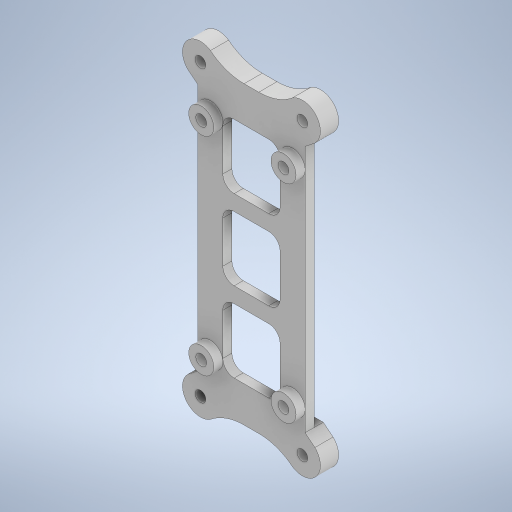
# Autodesk Inventor part: Flight Controller Mount
Saved by Autodesk Inventor 2023 (Build 270158000, 158)
## iProperties
Created: 2022-11-05
Part Number: Flight Controller Mount
Material: Generic
Document SubType Name: Modeling
Designer: mjlangfo
Density: 1 g/cm^3
Appearance: Default
Author: mjlangfo
Autodesk Inventor part; units mm, degrees
ref_plane "YZ Plane" through (0, 0, 0) normal (1, 0, 0) x (0, 1, 0)
ref_plane "XZ Plane" through (0, 0, 0) normal (0, 1, 0) x (-1, 0, 0)
ref_plane "XY Plane" through (0, 0, 0) normal (0, 0, 1) x (1, 0, 0)
sketch "Sketch1" plane through (0, 0, 0) normal (0, 0, 1) x (1, 0, 0)
  line L0 (28.2876, 87.8245) -> (13.6204, 76.0012) projected
  arc A0 (28.2876, 87.8245) -> (28.7404, 92.0429) centre (26.4048, 90.1602) ccw construction
  line L1 (26.2301, 95.1571) -> (28.7404, 92.0429) construction
  arc A1 (26.2301, 95.1571) -> (22.0117, 95.61) centre (23.8944, 93.2744) ccw construction
  line L2 (11.4653, 87.1085) -> (22.0117, 95.61) construction
  arc A2 (2.0515, 83.7867) -> (11.4653, 87.1085) centre (2.0515, 98.7867) ccw projected
  line L3 (-2.0515, 83.7867) -> (2.0515, 83.7867) projected
  arc A3 (-11.4653, 87.1085) -> (-2.0515, 83.7867) centre (-2.0515, 98.7867) ccw projected
  line L4 (-22.0117, 95.61) -> (-11.4653, 87.1085) construction
  arc A4 (-22.0117, 95.61) -> (-26.2301, 95.1571) centre (-23.8944, 93.2744) ccw construction
  line L5 (-28.7404, 92.0429) -> (-26.2301, 95.1571) construction
  arc A5 (-28.7404, 92.0429) -> (-28.2876, 87.8245) centre (-26.4048, 90.1602) ccw construction
  line L6 (-13.6204, 76.0012) -> (-28.2876, 87.8245) projected
  arc A6 (-13.6204, 76.0012) -> (-7.3445, 73.7867) centre (-7.3445, 83.7867) ccw construction
  line L7 (7.3445, 73.7867) -> (-7.3445, 73.7867) projected
  arc A7 (7.3445, 73.7867) -> (13.6204, 76.0012) centre (7.3445, 83.7867) ccw construction
  circle A8 centre (-23.5925, 90.4621) radius 1.475 construction
  circle A9 centre (23.5925, 90.4621) radius 1.475 construction
  circle A10 centre (-14.25, 82.931) radius 1.475 projected
  circle A11 centre (14.25, 82.931) radius 1.475 projected
  line L8 (28.2876, -2.9109) -> (13.6204, 8.9124) projected
  arc A12 (13.6204, 8.9124) -> (7.3445, 11.127) centre (7.3445, 1.127) ccw construction
  line L9 (7.3445, 11.127) -> (-7.3445, 11.127) projected
  arc A13 (-7.3445, 11.127) -> (-13.6204, 8.9124) centre (-7.3445, 1.127) ccw construction
  line L10 (-13.6204, 8.9124) -> (-28.2876, -2.9109) projected
  arc A14 (-28.2876, -2.9109) -> (-28.7404, -7.1293) centre (-26.4048, -5.2465) ccw construction
  line L11 (-28.7404, -7.1293) -> (-26.2301, -10.2435) construction
  arc A15 (-26.2301, -10.2435) -> (-22.0117, -10.6963) centre (-23.8944, -8.3607) ccw construction
  line L12 (-22.0117, -10.6963) -> (-11.4653, -2.1949) construction
  arc A16 (-2.0515, 1.127) -> (-11.4653, -2.1949) centre (-2.0515, -13.873) ccw projected
  line L13 (-2.0515, 1.127) -> (2.0515, 1.127) projected
  arc A17 (11.4653, -2.1949) -> (2.0515, 1.127) centre (2.0515, -13.873) ccw projected
  line L14 (11.4653, -2.1949) -> (22.0117, -10.6963) construction
  arc A18 (22.0117, -10.6963) -> (26.2301, -10.2435) centre (23.8944, -8.3607) ccw construction
  line L15 (26.2301, -10.2435) -> (28.7404, -7.1293) construction
  arc A19 (28.7404, -7.1293) -> (28.2876, -2.9109) centre (26.4048, -5.2465) ccw construction
  circle A20 centre (-23.5925, -5.5484) radius 1.475 construction
  circle A21 centre (23.5925, -5.5484) radius 1.475 construction
  circle A22 centre (-14.25, 1.9826) radius 1.475 projected
  circle A23 centre (14.25, 1.9826) radius 1.475 projected
  arc A24 (10.926, -1.78) -> (17.0347, 6.1601) centre (14.25, 1.9826) ccw
  line L16 (-8, 79.2868) -> (-15, 79.2868) construction
  line L17 (-15, 79.2868) -> (-15, 77.1134)
  line L18 (-15, 5.6268) -> (-8, 5.6268) construction
  line L19 (-8, 14.302) -> (-8, 25.952)
  line L20 (15, 79.2868) -> (8, 79.2868) construction
  line L21 (8, 70.6117) -> (8, 58.9617)
  line L22 (8, 5.6268) -> (15, 5.6268) construction
  line L23 (15, 5.6268) -> (15, 7.8003)
  arc A25 (17.0347, 6.1601) -> (10.926, -1.78) centre (14.25, 1.9826) ccw construction
  arc A26 (17.0347, 78.7535) -> (10.926, 86.6936) centre (14.25, 82.931) ccw
  arc A27 (-10.926, 86.6936) -> (-17.0347, 78.7535) centre (-14.25, 82.931) ccw
  arc A28 (-11.4653, -2.1949) -> (-17.7412, 5.5906) centre (-14.25, 1.9826) ccw construction
  arc A29 (10.926, 86.6936) -> (17.0347, 78.7535) centre (14.25, 82.931) ccw construction
  arc A30 (-17.0347, 78.7535) -> (-10.926, 86.6936) centre (-14.25, 82.931) ccw construction
  arc A31 (-17.7412, 5.5906) -> (-11.4653, -2.1949) centre (-14.25, 1.9826) ccw
  line L24 (0, 73.7867) -> (4.825, 73.7867)
  line L25 (0, 73.7867) -> (-4.825, 73.7867)
  line L26 (0, 11.127) -> (4.825, 11.127)
  line L27 (0, 11.127) -> (-4.825, 11.127)
  arc A32 (8, 70.6117) -> (4.825, 73.7867) centre (4.825, 70.6117) ccw
  arc A33 (-4.825, 73.7867) -> (-8, 70.6117) centre (-4.825, 70.6117) ccw
  arc A34 (4.825, 11.127) -> (8, 14.302) centre (4.825, 14.302) ccw
  arc A35 (-8, 14.302) -> (-4.825, 11.127) centre (-4.825, 14.302) ccw
  line L28 (-15, 77.1134) -> (-15, 7.8003)
  line L29 (-15, 7.8003) -> (-15, 5.6268)
  line L30 (15, 7.8003) -> (15, 77.1134)
  line L31 (15, 77.1134) -> (15, 79.2868)
  line L32 (4.825, 55.7867) -> (-4.825, 55.7867)
  line L33 (-8, 55.7867) -> (-8, 51.4568) construction
  line L34 (-4.825, 51.4568) -> (4.825, 51.4568)
  line L35 (8, 51.4568) -> (8, 55.7867)
  line L36 (4.825, 33.4568) -> (-4.825, 33.4568)
  line L37 (-8, 33.4568) -> (-8, 29.127) construction
  line L38 (-4.825, 29.127) -> (4.825, 29.127)
  line L39 (8, 29.127) -> (8, 33.4568) construction
  line L40 (8, 55.7867) -> (8, 51.4568) construction
  line L41 (8, 48.2818) -> (8, 36.6318)
  line L42 (-8, 58.9617) -> (-8, 70.6117)
  line L43 (-8, 51.4568) -> (-8, 55.7867)
  line L44 (-8, 36.6318) -> (-8, 48.2818)
  line L45 (-8, 29.127) -> (-8, 33.4568)
  line L46 (8, 33.4568) -> (8, 29.127)
  line L47 (8, 25.952) -> (8, 14.302)
  arc A36 (4.825, 55.7867) -> (8, 58.9617) centre (4.825, 58.9617) ccw
  arc A37 (-8, 58.9617) -> (-4.825, 55.7867) centre (-4.825, 58.9617) ccw
  arc A38 (8, 48.2818) -> (4.825, 51.4568) centre (4.825, 48.2818) ccw
  arc A39 (-4.825, 51.4568) -> (-8, 48.2818) centre (-4.825, 48.2818) ccw
  arc A40 (-8, 36.6318) -> (-4.825, 33.4568) centre (-4.825, 36.6318) ccw
  arc A41 (4.825, 33.4568) -> (8, 36.6318) centre (4.825, 36.6318) ccw
  arc A42 (8, 25.952) -> (4.825, 29.127) centre (4.825, 25.952) ccw
  arc A43 (-4.825, 29.127) -> (-8, 25.952) centre (-4.825, 25.952) ccw
  point P0 (0, 0)
  point P1 (0, 1.127)
  point P2 (0, 83.7867)
  point P3 (8, 73.8082)
  point P4 (15, 73.7867)
  point P5 (-15, 73.7867)
  point P6 (15, 11.127)
  point P7 (-15, 11.127)
  point P8 (-17.7412, 79.3231)
  point P9 (17.7412, 5.5906)
  point P10 (17.7412, 79.3231)
  point P11 (-4.825, 73.7867)
  point P12 (4.825, 73.7867)
  point P13 (4.825, 11.127)
  point P14 (-4.825, 11.127)
  point P15 (0, 33.4568)
  dimension "d0" = 7
  dimension "d1" = 7
  dimension "d2" = 73.66
  dimension "d5" = 4.4999
  dimension "d6" = 4.4999
  dimension "d9" = 3.175
  dimension "d10" = 3.175
  dimension "d16" = 30
  dimension "d17" = 15
  dimension "d32" = 18
  dimension "d33" = 18
  dimension "d34" = 18
  dimension "d35" = 4.3299
  dimension "d36" = 4.3299
  dimension "d37" = 3.175
  constraints: 64 end point, 49 point on line, 48 point on circle, 40 tangent, 36 parallel, 20 centre point, 10 perpendicular, 9 equal radius, 5 midpoint, 4 coincident, 3 horizontal
  measures "d0" distance of L20.start L20.end
  measures "d1" distance of L16.start L16.end
  measures "d2" distance of L18.end L16.start
  measures "d5" distance between parallel lines of L3 L20
  measures "d6" distance between parallel lines of L13 L22
  measures "d9" radius of A32
  measures "d10" radius of A34
  measures "d16" distance between parallel lines of L28 L30
  measures "d17" distance from line of point (0, 83.787) L28
  measures "d32" distance between parallel lines of L32 L24
  measures "d33" distance from line of point (0, 33.457) L34
  measures "d34" distance between parallel lines of L26 L38
  measures "d35" distance between parallel lines of L34 L32
  measures "d36" distance between parallel lines of L38 L36
  measures "d37" radius of A36
extrude "Extrusion1" add sketch "Sketch1" along normal blind 2.54 contours L0 L30 L8 A24 A17 L13 A16 A31 L10 L28 L6 A27 A3 L3 A2 A26
sketch "Sketch2" plane through (0, 0, 2.54) normal (0, 0, 1) x (1, 0, 0)
  line L0 (2.0515, 83.7867) -> (-2.0515, 83.7867) projected
  line L1 (-2.0515, 1.127) -> (2.0515, 1.127) projected
  line L2 (15, 7.8003) -> (15, 77.1134) projected
  line L3 (-15, 77.1134) -> (-15, 7.8003) projected
  circle A0 centre (11.5, 71.4568) radius 3.5
  circle A1 centre (11.5, 13.4568) radius 3.5
  circle A2 centre (-11.5, 13.4568) radius 3.5
  circle A3 centre (-11.5, 71.4568) radius 3.5
  point P0 (0, 0)
  point P1 (0, 83.7867)
  point P2 (0, 83.7867)
  point P3 (0, 83.7867)
  point P4 (0, 1.127)
  dimension "d13" = 7
  dimension "d14" = 58
  dimension "d15" = 23
  dimension "d18" = 7
  dimension "d19" = 7
  dimension "d20" = 7
  dimension "d22" = 23
  dimension "d23" = 58
  dimension "d24" = 11.5
  dimension "d27" = 12.3299
  dimension "d29" = 12.3299
  constraints: 4 centre point, 4 midpoint, 1 horizontal alignment, 1 vertical alignment
  measures "d13" diameter of A0
  measures "d14" distance of A1.centre A0.centre
  measures "d15" distance of A2.centre A1.centre
  measures "d18" diameter of A1
  measures "d19" diameter of A2
  measures "d20" diameter of A3
  measures "d22" distance of A3.centre A0.centre
  measures "d23" distance of A2.centre A3.centre
  measures "d24" horizontal distance of point (0, 83.787) A0.centre
  measures "d27" distance from line of L0 A0.centre
  measures "d29" distance from line of L1 A1.centre
extrude "Extrusion2" add sketch "Sketch2" along normal blind 2.54
sketch "Sketch3" plane through (-11.5, 71.4568, 5.08) normal (0, 0, 1) x (1, 0, 0)
  circle A0 centre (23, 0) radius 3.5 projected
  circle A1 centre (0, 0) radius 3.5 projected
  circle A2 centre (0, -58) radius 3.5 projected
  circle A3 centre (23, -58) radius 3.5 projected
  circle A4 centre (23, 0) radius 1.5
  circle A5 centre (0, 0) radius 1.5
  circle A6 centre (0, -58) radius 1.5
  circle A7 centre (23, -58) radius 1.5
  point P0 (11.5, -71.4568)
  dimension "d38" = 3
  dimension "d39" = 3
  dimension "d40" = 3
  dimension "d41" = 3
  constraints: 4 centre point, 4 coincident
  measures "d38" diameter of A4
  measures "d39" diameter of A5
  measures "d40" diameter of A6
  measures "d41" diameter of A7
extrude "Extrusion3" cut sketch "Sketch3" against normal up to next contours A4 | A5 | A6 | A7
sketch "Sketch4" plane through (0, 0, 0) normal (0, 0, -1) x (-1, 0, 0)
  line L0 (-15, 71.4568) -> (-15, 77.1134) projected
  line L1 (15, 77.1134) -> (-15, 77.1134)
  line L2 (15, 77.1134) -> (15, 7.8003) projected
  line L3 (-17.7412, 5.5906) -> (-15, 7.8003) projected
  line L4 (15, 7.8003) -> (-15, 7.8003)
  circle A0 centre (11.5, 13.4568) radius 1.5 projected
  circle A1 centre (-11.5, 13.4568) radius 1.5 projected
  circle A2 centre (11.5, 71.4568) radius 1.5 projected
  circle A3 centre (-11.5, 71.4568) radius 1.5 projected
  arc A4 (2.0515, 83.7867) -> (11.4653, 87.1085) centre (2.0515, 98.7867) ccw projected
  line L5 (-2.0515, 83.7867) -> (2.0515, 83.7867) projected
  arc A5 (-11.4653, 87.1085) -> (-2.0515, 83.7867) centre (-2.0515, 98.7867) ccw projected
  arc A6 (-11.4653, 87.1085) -> (-17.7412, 79.3231) centre (-14.25, 82.931) ccw projected
  line L6 (-15, 77.1134) -> (-17.7412, 79.3231) projected
  line L7 (-15, 7.8003) -> (-15, 77.1134) projected
  line L8 (-17.7412, 5.5906) -> (-15, 7.8003) projected
  arc A7 (-17.7412, 5.5906) -> (-11.4653, -2.1949) centre (-14.25, 1.9826) ccw projected
  arc A8 (-2.0515, 1.127) -> (-11.4653, -2.1949) centre (-2.0515, -13.873) ccw projected
  line L9 (2.0515, 1.127) -> (-2.0515, 1.127) projected
  arc A9 (11.4653, -2.1949) -> (2.0515, 1.127) centre (2.0515, -13.873) ccw projected
  arc A10 (11.4653, -2.1949) -> (17.7412, 5.5906) centre (14.25, 1.9826) ccw projected
  line L10 (15, 7.8003) -> (17.7412, 5.5906) projected
  line L11 (15, 77.1134) -> (15, 7.8003) projected
  line L12 (17.7412, 79.3231) -> (15, 77.1134) projected
  arc A11 (17.7412, 79.3231) -> (11.4653, 87.1085) centre (14.25, 82.931) ccw projected
  line L13 (8, 14.302) -> (8, 25.952) projected
  arc A12 (4.825, 11.127) -> (8, 14.302) centre (4.825, 14.302) ccw projected
  line L14 (-4.825, 11.127) -> (4.825, 11.127) projected
  arc A13 (-8, 14.302) -> (-4.825, 11.127) centre (-4.825, 14.302) ccw projected
  line L15 (-8, 25.952) -> (-8, 14.302) projected
  arc A14 (-4.825, 29.127) -> (-8, 25.952) centre (-4.825, 25.952) ccw projected
  line L16 (4.825, 29.127) -> (-4.825, 29.127) projected
  arc A15 (8, 25.952) -> (4.825, 29.127) centre (4.825, 25.952) ccw projected
  line L17 (-8, 70.6117) -> (-8, 58.9617) projected
  arc A16 (-4.825, 73.7867) -> (-8, 70.6117) centre (-4.825, 70.6117) ccw projected
  line L18 (4.825, 73.7867) -> (-4.825, 73.7867) projected
  arc A17 (8, 70.6117) -> (4.825, 73.7867) centre (4.825, 70.6117) ccw projected
  line L19 (8, 58.9617) -> (8, 70.6117) projected
  arc A18 (4.825, 55.7867) -> (8, 58.9617) centre (4.825, 58.9617) ccw projected
  line L20 (-4.825, 55.7867) -> (4.825, 55.7867) projected
  arc A19 (-8, 58.9617) -> (-4.825, 55.7867) centre (-4.825, 58.9617) ccw projected
  line L21 (8, 36.6318) -> (8, 48.2818) projected
  arc A20 (4.825, 33.4568) -> (8, 36.6318) centre (4.825, 36.6318) ccw projected
  line L22 (-4.825, 33.4568) -> (4.825, 33.4568) projected
  arc A21 (-8, 36.6318) -> (-4.825, 33.4568) centre (-4.825, 36.6318) ccw projected
  line L23 (-8, 48.2818) -> (-8, 36.6318) projected
  arc A22 (-4.825, 51.4568) -> (-8, 48.2818) centre (-4.825, 48.2818) ccw projected
  line L24 (4.825, 51.4568) -> (-4.825, 51.4568) projected
  arc A23 (8, 48.2818) -> (4.825, 51.4568) centre (4.825, 48.2818) ccw projected
  circle A24 centre (-14.25, 1.9826) radius 1.475 projected
  circle A25 centre (14.25, 1.9826) radius 1.475 projected
  circle A26 centre (-14.25, 82.931) radius 1.475 projected
  circle A27 centre (14.25, 82.931) radius 1.475 projected
  point P0 (0, 0)
  point P1 (-17.7412, 5.5906)
  constraints: 4 end point, 2 horizontal
extrude "Extrusion4" add sketch "Sketch4" along normal blind 2.54 contours L6 A6 A5 L5 A4 A11 L12 L1 | L4 L10 A10 A9 L9 A8 A7 L3
equation "\"d1\" = d0"
equation "\"d5\" = d6"
equation "\"d17\" = 0.5 * d16"
equation "\"d32\" = d33"
equation "\"d34\" = d33"
equation "\"d35\" = d36"
equation "\"d18\" = d13"
equation "\"d19\" = d13"
equation "\"d20\" = d13"
equation "\"d22\" = d15"
equation "\"d23\" = d14"
equation "\"d24\" = 0.5 * d22"
equation "\"d27\" = d29"
equation "\"d39\" = d38"
equation "\"d40\" = d38"
equation "\"d41\" = d38"
body "Solid1"
